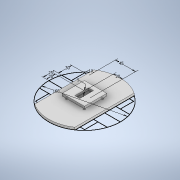
# Autodesk Inventor part: Bellamy-cialo_glowne
Saved by Autodesk Inventor 2020 (Build 240168000, 168)
## iProperties
Created: 2022-12-15
Part Number: Bellamy-cialo_glowne
Material: Ogólny
Document SubType Name: Modeling
Designer: User
Density: 1 g/cm^3
Appearance: Domyślna
Author: User
Autodesk Inventor part; units mm, degrees
ref_plane "YZ Plane" through (0, 0, 0) normal (1, 0, 0) x (0, 1, 0)
ref_plane "XZ Plane" through (0, 0, 0) normal (0, 1, 0) x (-1, 0, 0)
ref_plane "XY Plane" through (0, 0, 0) normal (0, 0, 1) x (1, 0, 0)
sketch "Szkic1" plane through (0, 0, 0) normal (0, 1, 0) x (-1, 0, 0)
  circle A0 centre (0, 0) radius 80
  line L0 (55, -25) -> (45, -25)
  line L1 (45, -25) -> (45, -55)
  line L2 (45, -55) -> (55, -55)
  line L3 (55, -55) -> (55, -25)
  line L4 (55, 25) -> (45, 25)
  line L5 (45, 25) -> (45, 55)
  line L6 (45, 55) -> (55, 55)
  line L7 (55, 55) -> (55, 25)
  line L8 (80, 0) -> (-80, 0)
  line L9 (0, 80) -> (0, -80)
  line L10 (-45, -25) -> (-55, -25)
  line L11 (-55, -25) -> (-55, -55)
  line L12 (-55, -55) -> (-45, -55)
  line L13 (-45, -55) -> (-45, -25)
  line L14 (-45, 55) -> (-55, 55)
  line L15 (-55, 55) -> (-55, 25)
  line L16 (-55, 25) -> (-45, 25)
  line L17 (-45, 25) -> (-45, 55)
  circle A1 centre (20, -20) radius 2.5
  circle A2 centre (20, 20) radius 2.5
  circle A3 centre (-20, -20) radius 2.5
  circle A4 centre (-20, 20) radius 2.5
  line L18 (45, -55) -> (45, -66.1438)
  line L19 (55, -25) -> (75.9934, -25)
  line L20 (45, 55) -> (45, 66.1438)
  line L21 (55, 25) -> (75.9934, 25)
  line L22 (-45, -55) -> (-45, -66.1438)
  line L23 (-55, -25) -> (-75.9934, -25)
  line L24 (-55, 25) -> (-75.9934, 25)
  line L25 (-45, 55) -> (-45, 66.1438)
  line L26 (45, -25) -> (45, 25)
  line L27 (-45, -25) -> (-45, 25)
  dimension "d0" = 160
  dimension "d1" = 10
  dimension "d2" = 30
  dimension "d3" = 25
  dimension "d4" = 45
  dimension "d5" = 5
  dimension "d6" = 20
  dimension "d7" = 20
  constraints: 56 end point, 9 symmetric about line, 8 parallel, 6 perpendicular, 6 point on circle, 5 centre point, 5 horizontal, 2 midpoint, 1 coincident, 1 collinear, 1 vertical, 16 other
  measures "d0" diameter of A0
  measures "d1" distance of L1.end L2.end
  measures "d2" distance of L2.end L0.start
  measures "d3" distance between parallel lines of L0 L8
  measures "d4" distance between parallel lines of L1 L9
  measures "d5" diameter of A1
  measures "d6" distance from line of L9 A1.centre
  measures "d7" distance from line of L8 A1.centre
extrude "Wyciągnięcie proste1" add sketch "Szkic1" along normal blind 5 contours L26 L1 L18 A0 L9 L8 | L8 L9 A0 L20 L5 L26 | L9 A0 L22 L13 L27 L8 | L8 L27 L17 L25 A0 L9
extrude "Wyciągnięcie proste2" add sketch "Szkic1" along normal blind 10 contours A1 | A2 | A3 | A4
fillet "Zaokrąglenie1" radius 2 1 edges at (0, 0, -80)
sketch "Sketch3" plane through (20, 10, 20) normal (0, 1, 0) x (1, 0, 0)
  line L0 (5, -5) -> (-45, -5)
  line L1 (-45, -5) -> (-45, 45)
  line L2 (-45, 45) -> (5, 45)
  line L3 (5, 45) -> (5, -5)
  circle A0 centre (-40, 0) radius 2.5 projected
  line L4 (-40, 0) -> (-40, -5)
  line L5 (-40, 0) -> (-45, 0)
  line L6 (-15.243, 4.7) -> (-26.243, 4.7)
  line L7 (-26.243, 4.7) -> (-26.243, 35.3)
  line L8 (-26.243, 35.3) -> (-15.243, 35.3)
  line L9 (-15.243, 35.3) -> (-15.243, 4.7)
  line L10 (-20.743, 4.7) -> (-20.743, -5)
  circle A1 centre (0, 0) radius 2.5 projected
  line L11 (0, 0) -> (-15.243, 4.7)
  point P0 (-20, 20)
  dimension "d30" = 50
  dimension "d31" = 50
  dimension "d34" = 5
  dimension "d35" = 5
  dimension "d36" = 30.6
  dimension "d37" = 11
  dimension "d38" = 9.7
  dimension "d40" = 15.243
  constraints: 24 end point, 5 parallel, 4 perpendicular, 3 point on line, 2 horizontal, 1 midpoint
  measures "d30" distance of L0.start L0.end
  measures "d31" distance of L0.end L1.end
  measures "d34" distance of L4.start L4.end
  measures "d35" distance of L4.start L5.end
  measures "d36" distance of L8.end L6.start
  measures "d37" distance of L6.start L6.end
  measures "d38" distance of L10.start L10.end
  measures "d40" horizontal distance of L11.start L6.start
extrude "Extrusion4" add sketch "Sketch3" along normal blind 5 contours L0 L4 A0 L5 L1 L2 L3 | L0 L1 L5 A0 L4 | L4 L5 A0 | A0 L5 L4 | A1
sketch "Sketch4" plane through (25, 10, 25) normal (1, 0, 0) x (0, 0, -1)
  circle A0 centre (38.5, 2.5) radius 1.4929
  line L0 (50, 0) -> (50, 5) projected
  line L1 (0, 0) -> (50, 0) projected
  point P0 (25, -10)
  dimension "d43" = 11.5
  dimension "d44" = 2.5
  constraints: 1 centre point
  measures "d43" distance from line of L0 A0.centre
  measures "d44" distance from line of L1 A0.centre
hole "Hole2" at (25, 12.5, -13.5) direction (-1, 0, 0) diameter 3 depth 3
sketch "Sketch5" plane through (-25, 10, -25) normal (-1, 0, 0) x (0, 0, 1)
  circle A0 centre (11.5, 2.5) radius 1.5 projected
  circle A1 centre (11.5, 2.5) radius 1.5
  point P0 (25, -10)
  constraints: 1 centre point, 1 coincident
hole "Hole3" at (-25, 12.5, -13.5) direction (1, 0, 0) diameter 3 depth 3
sketch "Sketch6" plane through (-25, 10, 25) normal (0, 0, 1) x (1, 0, 0)
  circle A0 centre (11, 2.5) radius 1.755
  line L0 (0, 0) -> (0, 5) projected
  line L1 (0, 0) -> (50, 0) projected
  point P0 (25, -10)
  dimension "d59" = 11
  dimension "d60" = 2.5
  constraints: 1 centre point
  measures "d59" distance from line of A0.centre L0
  measures "d60" distance from line of L1 A0.centre
hole "Hole4" at (-14, 12.5, 25) direction (0, 0, -1) diameter 3 depth 3
sketch "Sketch7" plane through (25, 10, -25) normal (0, 0, -1) x (-1, 0, 0)
  circle A0 centre (45, 2.5) radius 0.9964
  line L0 (0, 0) -> (50, 0) projected
  line L1 (50, 0) -> (50, 5) projected
  line L2 (25, 0) -> (25, 5)
  circle A1 centre (5, 2.5) radius 0.9964
  line L3 (0, 0) -> (0, 5) projected
  point P0 (25, -10)
  dimension "d68" = 2.5
  dimension "d78" = 40
  dimension "d79" = 5
  dimension "d80" = 5
  constraints: 2 centre point, 2 end point, 1 midpoint, 1 vertical
  measures "d68" distance from line of A0.centre L0
  measures "d78" distance of A0.centre A1.centre
  measures "d79" distance from line of L3 A1.centre
  measures "d80" distance from line of L1 A0.centre
hole "Hole5" at (-20, 12.5, -25) at (20, 12.5, -25) direction (0, 0, 1) diameter 1.5 depth 2.5
